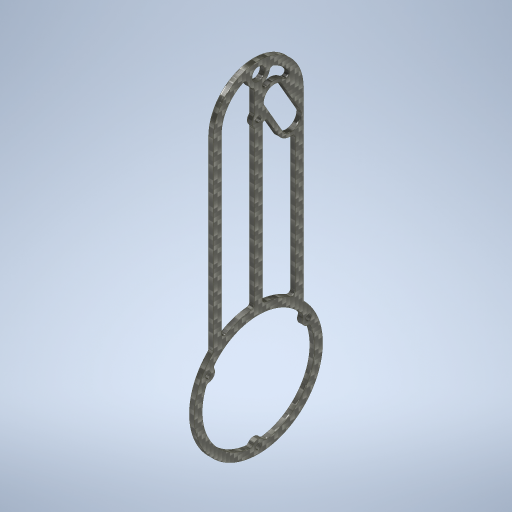
# Autodesk Inventor part: LowerArmFrame
Saved by Autodesk Inventor 2024.2 (Build 282272000, 272)
## iProperties
Created: 2024-01-18
Part Number: LowerArmFrame
Material: CFRP
Document SubType Name: Modeling
Designer: Masato Kubotera
Density: 1.43 g/cm^3
Appearance: Carbon Fiber 1
Mass: 9.5835 g
Surface Area: 85.4471 cm^2
Volume: 6.70175 cm^3
Vendor: ALLPCB
Author: Masato Kubotera
Autodesk Inventor part; units mm, degrees
ref_plane "YZ Plane" through (0, 0, 0) normal (1, 0, 0) x (0, 1, 0)
ref_plane "XZ Plane" through (0, 0, 0) normal (0, 1, 0) x (-1, 0, 0)
ref_plane "XY Plane" through (0, 0, 0) normal (0, 0, 1) x (1, 0, 0)
sketch "Sketch1" plane through (0, 0, 0) normal (0, 1, 0) x (-1, 0, 0)
  line L0 (-28, -21) -> (-28, -135.6061)
  line L1 (0, 0) -> (0, -205) construction
  arc A0 (-28.5714, -137.0058) -> (28.5714, -137.0058) centre (0, -165) ccw
  line L2 (28, -21) -> (28, -135.6061)
  circle A1 centre (0, 0) radius 4 construction
  line L3 (0, 0) -> (20, -34.641) construction
  circle A2 centre (10, -17.3205) radius 20 construction
  circle A3 centre (0, 0) radius 40 construction
  arc A4 (17.3769, -38.8977) -> (24.9979, -34.4977) centre (20, -34.641) ccw construction
  arc A5 (15.9891, -40.194) -> (26.8144, -33.944) centre (20, -34.641) ccw
  line L4 (17.3769, -38.8977) -> (5.0021, -17.4638) construction
  line L5 (15.9891, -40.194) -> (3.1856, -18.0175)
  line L6 (24.9979, -34.4977) -> (12.6231, -13.0638) construction
  line L7 (26.8144, -33.944) -> (14.0109, -11.7675)
  line L8 (11.1895, -28.1808) -> (18.8105, -23.7808) construction
  arc A6 (12.6231, -13.0638) -> (5.0021, -17.4638) centre (10, -17.3205) ccw construction
  arc A7 (14.0109, -11.7675) -> (3.1856, -18.0175) centre (10, -17.3205) ccw
  line L9 (0, 0) -> (20, 0) construction
  line L10 (20, 0) -> (40, 0) construction
  circle A8 centre (0, -165) radius 36 construction
  line L11 (0, -165) -> (-34.641, -145) construction
  line L12 (0, -165) -> (34.641, -145) construction
  arc A9 (28, -21) -> (-28, -21) centre (0, -21) ccw
  line L13 (-23, -128.6269) -> (-23, -21)
  line L14 (-2.5, -28.4686) -> (-2.5, -123.2418)
  arc A10 (-4.2857, -125.2303) -> (-20, -130.359) centre (0, -165) ccw
  line L15 (23, -128.6269) -> (23, -45.5955)
  line L16 (2.5, -28.4686) -> (2.5, -123.2418)
  arc A11 (20, -130.359) -> (4.2857, -125.2303) centre (0, -165) ccw
  arc A12 (12.2058, -39.141) -> (20.8182, -43.6037) centre (20, -34.641) ccw
  line L17 (12.2058, -39.141) -> (5.7488, -27.9571)
  arc A13 (-9.6282, -0.1122) -> (-23, -21) centre (0, -21) ccw
  arc A14 (-6.8374, -1.5) -> (-3.5, -6.0622) centre (0, 0) ccw
  arc A15 (15.9671, -10.583) -> (5.5, -9.5263) centre (10, -17.3205) ccw
  arc A16 (3.5, -6.0622) -> (6.8374, -1.5) centre (0, 0) ccw
  arc A17 (18.9401, -7.9511) -> (9.6282, -0.1122) centre (0, -21) ccw
  circle A18 centre (0, -24.5) radius 4 construction
  arc A19 (-23, -128.6269) -> (-20, -130.359) centre (-21, -128.6269) ccw
  arc A20 (-4.2857, -125.2303) -> (-2.5, -123.2418) centre (-4.5, -123.2418) ccw
  arc A21 (-2.5, -7.7942) -> (-3.5, -6.0622) centre (-4.5, -7.7942) ccw
  arc A22 (-6.8374, -1.5) -> (-9.6282, -0.1122) centre (-8.7909, -1.9286) ccw
  arc A23 (9.6282, -0.1122) -> (6.8374, -1.5) centre (8.7909, -1.9286) ccw
  arc A24 (15.9671, -10.583) -> (18.9401, -7.9511) centre (17.2931, -9.0858) ccw
  arc A25 (5.7488, -27.9571) -> (2.6778, -27.4714) centre (4.0167, -28.9571) ccw
  arc A26 (2.5, -123.2418) -> (4.2857, -125.2303) centre (4.5, -123.2418) ccw
  arc A27 (20, -130.359) -> (23, -128.6269) centre (21, -128.6269) ccw
  arc A28 (23, -45.5955) -> (20.8182, -43.6037) centre (21, -45.5955) ccw
  arc A29 (-3, -21.8542) -> (-3, -27.1458) centre (0, -24.5) ccw
  line L18 (-2.5, -7.7942) -> (-2.5, -20.5314)
  arc A30 (-2.5, -28.4686) -> (-3, -27.1458) centre (-4.5, -28.4686) ccw
  arc A31 (-3, -21.8542) -> (-2.5, -20.5314) centre (-4.5, -20.5314) ccw
  arc A32 (-32.037, -150.9064) -> (-28.2239, -144.3019) centre (-31.1769, -147) ccw
  arc A33 (3.8131, -199.7917) -> (-3.8131, -199.7917) centre (0, -201) ccw
  arc A34 (-32.037, -150.9064) -> (-3.8131, -199.7917) centre (0, -165) ccw
  arc A35 (28.2239, -144.3019) -> (32.037, -150.9064) centre (31.1769, -147) ccw
  arc A36 (3.8131, -199.7917) -> (32.037, -150.9064) centre (0, -165) ccw
  arc A37 (28.2239, -144.3019) -> (-28.2239, -144.3019) centre (0, -165) ccw
  arc A38 (-28.5714, -137.0058) -> (-28, -135.6061) centre (-30, -135.6061) ccw
  arc A39 (28, -135.6061) -> (28.5714, -137.0058) centre (30, -135.6061) ccw
  line L19 (2.5, -7.7942) -> (2.5, -7.7942)
  arc A40 (3.5, -6.0622) -> (2.5, -7.7942) centre (4.5, -7.7942) ccw
  arc A41 (2.5, -7.7942) -> (5.5, -9.5263) centre (4.5, -7.7942) ccw
  arc A42 (3, -27.1458) -> (2.6778, -27.4714) centre (0, -24.5) ccw
  arc A43 (3, -27.1458) -> (2.5, -28.4686) centre (4.5, -28.4686) ccw
  point P0 (-28, -136.4343)
  point P1 (28, -136.4343)
  point P2 (30, -113.5425)
  point P3 (15.9891, -40.194)
  point P4 (-14.0109, -11.7675)
  point P5 (0, 7)
  point P6 (-23, -132.2739)
  point P7 (-2.5, -125.0782)
  point P8 (23, -132.2739)
  point P9 (2.5, -125.0782)
  point P10 (23, -43.1263)
  point P11 (-2, -6.7082)
  point P12 (25.7858, -19.6697)
  point P13 (-2.5, -21.3775)
  point P14 (-1.5, -28.2081)
  point P15 (-27.7128, -149)
  point P16 (27.7128, -149)
  point P17 (2.5, -7.7942)
  point P18 (2.8577, -27.3272)
  dimension "d1" = 205
  dimension "d2" = 80
  dimension "d3" = 8
  dimension "d15" = 8.8
  dimension "d16" = 12.5
  dimension "d17" = 10
  dimension "d18" = 1.85
  dimension "d19" = 1.85
  dimension "d20" = 60
  dimension "d21" = 20
  dimension "d22" = 20
  dimension "d24" = 20
  dimension "d29" = 30
  dimension "d31" = 72
  dimension "d32" = 120
  dimension "d40" = 7
  dimension "d41" = 56
  dimension "d43" = 24.5
  dimension "d44" = 5
  dimension "d46" = 5
  dimension "d50" = 8
  dimension "d52" = 2
  dimension "d54" = 5
  dimension "d57" = 9
  dimension "d58" = 8
  constraints: 106 point on circle, 44 centre point, 41 end point, 34 tangent, 22 symmetric about line, 20 coincident, 19 equal radius, 17 point on line, 5 vertical, 3 midpoint, 3 parallel, 2 collinear, 11 other
  measures "d1" distance of L1.start L1.end
  measures "d2" diameter of A0
  measures "d3" diameter of A1
  measures "d15" distance between parallel lines of L6 L4
  measures "d16" distance between parallel lines of L5 L7
  measures "d17" diameter of A4
  measures "d18" distance between parallel lines of L7 L6
  measures "d19" radial gap between concentric circles of A5 A4
  measures "d20" angle of L3 L9
  measures "d21" distance of L9.end L10.end
  measures "d22" radius of A2
  measures "d24" distance of L3.end A6.centre
  measures "d29" angle of L3 L1
  measures "d31" diameter of A8
  measures "d32" angle of L1 L11
  measures "d40" distance of point (0, 7) L3.start
  measures "d41" distance between parallel lines of L0 L2
  measures "d43" distance of point (0, -24.5) point (0, 0)
  measures "d44" distance between parallel lines of L0 L13
  measures "d46" distance between parallel lines of L16 L14
  measures "d50" diameter of A18
  measures "d52" radius of A19
  measures "d54" radial gap between concentric circles of A0 A34
  measures "d57" radius of A12
  measures "d58" diameter of A32
extrude "Extrusion1" add sketch "Sketch1" along normal blind 3 contours A9 L2 A39 A0 A38 L0 | A29 A42 A43 A25
hole "Phi8.0-H7" at (0, 0, 0) direction (0, 1, 0) diameter 8 end through all
hole "Phi3.5" at (31.1769, 0, -147) at (-31.1769, 0, -147) at (0, 0, -201) at (0, 0, -24.5) direction (0, 1, 0) diameter 3.5 end through all
fillet "R2" radius 2 10 edges at (-3.1856, 1.5, -18.0175) (-14.0109, 1.5, -11.7675) (-26.8144, 1.5, -33.944) (-15.9891, 1.5, -40.194) (32.037, 1.5, -150.9064) (-32.037, 1.5, -150.9064) (-3.8131, 1.5, -199.7917) (3.8131, 1.5, -199.7917) (28.2239, 1.5, -144.3019) (-28.2239, 1.5, -144.3019)
equation "\"d19\" = d18"
equation "\"d24\" = d21"
equation "\"d13\" = d5"
equation "\"d5\" = 8.1"
body "Solid1"
